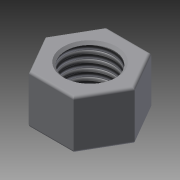
# Autodesk Inventor part: 砂轮架带动曲柄轴盖螺帽
Saved by Autodesk Inventor 2015 (Build 190159000, 159)
## iProperties
Created: 2017-05-17
Part Number: 砂轮架带动曲柄轴盖螺帽
Material: 常规
Document SubType Name: Modeling
Designer: Administrator
Density: 1 g/cm^3
Appearance: 默认
Author: Administrator
Autodesk Inventor part; units mm, degrees
ref_plane "YZ Plane" through (0, 0, 0) normal (1, 0, 0) x (0, 1, 0)
ref_plane "XZ Plane" through (0, 0, 0) normal (0, 1, 0) x (-1, 0, 0)
ref_plane "XY Plane" through (0, 0, 0) normal (0, 0, 1) x (1, 0, 0)
sketch "草图1" plane through (0, 0, 0) normal (0, 0, 1) x (1, 0, 0)
  circle A0 centre (0, 0) radius 2.5
  line L0 (2.3094, -4) -> (-2.3094, -4)
  line L1 (-2.3094, -4) -> (-4.6188, 0)
  line L2 (-4.6188, 0) -> (-2.3094, 4)
  line L3 (-2.3094, 4) -> (2.3094, 4)
  line L4 (2.3094, 4) -> (4.6188, 0)
  line L5 (4.6188, 0) -> (2.3094, -4)
  line L6 (0, 0) -> (0, 1.5398)
  point P0 (0, 4)
  dimension "d0" = 5
  dimension "d1" = 1.5398
  dimension "d2" = 8
  constraints: 14 end point, 2 coincident, 1 centre point, 1 midpoint, 1 point on line, 1 vertical, 13 other
  measures "d0" diameter of A0
  measures "d1" distance of L6.start L6.end
  measures "d2" distance between parallel lines of L0 L3
extrude "拉伸1" add sketch "草图1" along normal blind 5
thread "螺纹1" size "M5x0.8" class "6H" standard "ANSI Metric M Profile" full length
fillet "圆角1" radius 0.25 12 edges at (0, 4, 5) (3.4641, 2, 5) (3.4641, -2, 5) (-3.4641, -2, 5) (-3.4641, 2, 5) (0, -4, 5) (3.4641, -2, 0) (3.4641, 2, 0) (0, 4, 0) (-3.4641, 2, 0) (-3.4641, -2, 0) (0, -4, 0)
chamfer "倒角1" distance 0.25 angle 45 2 edges at (-2.5, 0, 5) (-2.5, 0, 0)
